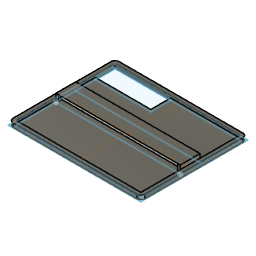
Center Side Low Cover 1x1 v4 (Autodesk Fusion 360 design; units mm, degrees)
Autodesk Fusion 360 part; units mm, degrees
sketch "Schizzo1" plane through (0, 0, 0) normal (0, 0, 1) x (1, 0, 0)
  line L0 (-42.5691, 59.0067) -> (24.1309, 59.0067) construction
  line L1 (24.1309, 59.0067) -> (24.1309, 5.3067) construction
  line L2 (24.1309, 5.3067) -> (-42.5691, 5.3067) construction
  line L3 (-42.5691, 5.3067) -> (-42.5691, 59.0067) construction
  line L4 (24.0309, 58.9067) -> (24.0309, 5.4067)
  line L5 (24.0309, 5.4067) -> (-42.4691, 5.4067)
  line L6 (-42.4691, 5.4067) -> (-42.4691, 58.9067)
  line L7 (-42.4691, 58.9067) -> (24.0309, 58.9067)
  line L8 (22.1309, 7.3067) -> (-40.5691, 7.3067)
  line L9 (-40.5691, 7.3067) -> (-40.5691, 57.0067)
  line L10 (-40.5691, 57.0067) -> (22.1309, 57.0067)
  line L11 (22.1309, 57.0067) -> (22.1309, 7.3067)
  line L12 (-40.5691, 57.0067) -> (-12.5691, 57.0067)
  line L13 (-12.5691, 57.0067) -> (-12.5691, 47.0067)
  line L14 (-12.5691, 47.0067) -> (-40.5691, 47.0067)
  line L15 (-40.5691, 47.0067) -> (-40.5691, 57.0067)
  line L16 (-42.5691, 32.1567) -> (24.1309, 32.1567) construction
  line L17 (-9.2191, 59.0067) -> (-9.2191, 5.3067) construction
  line L18 (-40.5691, 37.1567) -> (22.1309, 37.1567)
  line L19 (-40.5691, 27.1567) -> (22.1309, 27.1567)
  dimension "d1" = 66.7
  dimension "d2" = 53.7
  dimension "d3" = 0.1
  dimension "d8" = 2
  dimension "d9" = 28
  dimension "d10" = 10
  dimension "d11" = 10
  constraint horizontal L0
  constraint vertical L1
  constraint horizontal L2
  constraint vertical L3
  constraint horizontal L12
  constraint vertical L13
  constraint horizontal L14
  constraint vertical L15
  constraint midpoint L3 L16.start
  constraint midpoint L1 L16.end
  constraint midpoint L0 L17.start
  constraint midpoint L2 L17.end
  constraint coincident L9 L18.start
  constraint coincident L11 L18.end
  constraint perpendicular L11 L18
  constraint symmetric L16 L18.start L19.start
  constraint symmetric L16 L18.end L19.end
  measures "d1" distance of L0.start L0.end
  measures "d2" distance of L0.start L2.end
  measures "d9" distance of L9.end L12.end
  measures "d10" distance of L9.end L14.end
  measures "d11" distance of L18 L19
extrude "Estrusione1" add sketch "Schizzo1" along normal blind 4 contours L8 L9 L11 L19 | L9 L11 L18 L19 | L9 L10 L11 L13 L14 L18
extrude "Estrusione4" add sketch "Schizzo1" along normal blind 2
fillet "Raccordo1" radius 2 4 edges at (-42.4691, 5.4067, 1) (24.0309, 5.4067, 1) (24.0309, 58.9067, 1) (-42.4691, 58.9067, 1)
extrude "Estrusione2" cut sketch "Schizzo1" against normal blind 3 from surface at 4 contours L8 L9 L11 L19 | L9 L10 L11 L13 L14 L18
ref_plane "Piano di lavoro1" through (-9.2191, 32.1567, 0) normal (1, 0, 0) x (0, -1, 0)
sketch "Schizzo2" plane through (-9.2191, 0, 0) normal (1, 0, 0) x (0, 1, 0)
  line L0 (5.4067, 4) -> (58.9067, 4) construction
  line L1 (58.9067, 4) -> (58.9067, 0) construction
  line L2 (58.9067, 0) -> (5.4067, 0) construction
  line L3 (5.4067, 0) -> (5.4067, 4) construction
  line L4 (58.9067, 2) -> (58.9067, 0) construction
  line L5 (7.4067, 0) -> (56.9067, 0) construction
  line L6 (5.4067, 0) -> (5.4067, 2) construction
  line L7 (37.1567, 4) -> (27.1567, 4) construction
  line L8 (32.1567, 4) -> (32.1567, 0) construction
  line L9 (27.1567, 4) -> (27.1567, 0) construction
  line L10 (27.1567, 2) -> (27.1567, 4) construction
  line L11 (5.4067, 1) -> (58.9067, 1) construction
  line L12 (7.3067, 1) -> (27.1567, 1) construction
  line L13 (37.1567, 4) -> (37.1567, 0) construction
  line L14 (27.1567, 4) -> (28.8887, 1)
  line L15 (27.1567, 4) -> (30.6208, 4) construction
  line L16 (28.8887, 1) -> (27.1567, 1)
  line L17 (27.1567, 1) -> (27.1567, 4)
  line L18 (37.1567, 4) -> (35.4246, 1)
  line L19 (37.1567, 1) -> (37.1567, 4)
  line L20 (35.4246, 1) -> (37.1567, 1)
  dimension "d24" = 60
  constraint horizontal L0
  constraint vertical L1
  constraint horizontal L2
  constraint vertical L3
  constraint collinear L1 L4
  constraint collinear L2 L5
  constraint collinear L3 L6
  constraint collinear L0 L7
  constraint midpoint L7 L8.start
  constraint midpoint L5 L8.end
  constraint coincident L0 L7.end
  constraint coincident L5 L9.end
  constraint collinear L9 L10
  constraint coincident L3 L11.start
  constraint coincident L1 L11.end
  constraint perpendicular L1 L11
  constraint collinear L11 L12
  constraint symmetric L8 L7.end L7.start
  constraint symmetric L8 L9.end L13.end
  constraint horizontal L15
  constraint coincident L7.end L9.start
  constraint coincident L11 L14.end
  constraint coincident L12.end L16.end
  constraint symmetric L8 L14.end L18.end
  constraint symmetric L8 L12.end L19.start
  measures "d24" angle of L14 L15
extrude "Estrusione3" cut sketch "Schizzo2" along normal mid plane 60
